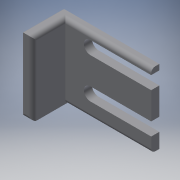
# Autodesk Inventor part: Pusher
Saved by Autodesk Inventor 2019.3 (Build 233278000, 278)
## iProperties
Created: 2020-09-18
Part Number: Pusher
Material: Generisch
Document SubType Name: Modeling
Designer: Nicolas Frick
Density: 1 g/cm^3
Appearance: Vorgabe
Author: Nicolas Frick
Autodesk Inventor part; units mm, degrees
ref_plane "YZ Plane" through (0, 0, 0) normal (1, 0, 0) x (0, 1, 0)
ref_plane "XZ Plane" through (0, 0, 0) normal (0, 1, 0) x (-1, 0, 0)
ref_plane "XY Plane" through (0, 0, 0) normal (0, 0, 1) x (1, 0, 0)
sketch "Skizze1" plane through (0, 0, 0) normal (0, 0, 1) x (1, 0, 0)
  line L0 (18, 18) -> (18, 0) construction
  line L1 (2, 18) -> (18, 18) construction
  line L2 (2, 0) -> (2, 18) construction
  line L3 (18, 0) -> (2, 0) construction
  line L4 (2, 18) -> (18, 18)
  line L5 (18, 0) -> (2, 0)
  line L6 (0.5764, 6.9713) -> (-2.7403, -18.928) construction
  circle A0 centre (14.2155, 15.0333) radius 1.2952 construction
  circle A1 centre (14.2155, 5.2246) radius 1.25 construction
  line L7 (2, 18) -> (-5.9127, 18)
  line L8 (-5.9127, 18) -> (-5.9127, 0)
  line L9 (-5.9127, 0) -> (2, 0)
  line L10 (18, 15.0333) -> (3.145, 15.0333) construction
  line L11 (18, 16.6333) -> (3.145, 16.6333)
  line L12 (3.145, 13.4333) -> (18, 13.4333)
  arc A2 (3.145, 16.6333) -> (3.145, 13.4333) centre (3.145, 15.0333) ccw
  line L13 (18, 5.2246) -> (3.145, 5.2246) construction
  line L14 (18, 6.8246) -> (3.145, 6.8246)
  line L15 (3.145, 3.6246) -> (18, 3.6246)
  arc A3 (3.145, 6.8246) -> (3.145, 3.6246) centre (3.145, 5.2246) ccw
  line L16 (-5.9127, 18) -> (18, 18)
  line L17 (18, 0) -> (-5.9127, 0)
  line L18 (-5.9127, 0) -> (-5.9127, 18)
  line L19 (18, 16.6333) -> (3.145, 16.6333)
  line L20 (18, 13.4333) -> (3.145, 13.4333)
  line L21 (18, 6.8246) -> (3.145, 6.8246)
  line L22 (18, 3.6246) -> (3.145, 3.6246)
  line L23 (18, 18) -> (18, 16.6333)
  line L24 (18, 18) -> (18, 16.6333)
  line L25 (18, 13.4333) -> (18, 6.8246)
  line L26 (18, 3.6246) -> (18, 0)
  line L27 (18, 13.4333) -> (18, 6.8246)
  line L28 (18, 3.6246) -> (18, 0)
  point P0 (0, 0)
  point P1 (10.5725, 15.0333)
  point P2 (10.5725, 5.2246)
  dimension "d0" = 2.5
  dimension "d1" = 3.2
  dimension "d2" = 3.2
  constraints: 52 end point, 11 perpendicular, 8 parallel, 4 centre point, 4 point on circle, 4 tangent, 3 collinear, 3 horizontal, 2 midpoint, 1 point on line
  measures "d0" diameter of A1
  measures "d1" diameter of A2
  measures "d2" diameter of A3
extrude "Extrusion1" add sketch "Skizze1" along normal blind 10
sketch "Skizze2" plane through (0, 0, 10) normal (0, 0, 1) x (1, 0, 0)
  line L0 (-5.9127, 0) -> (18, 0) construction
  line L1 (18, 0) -> (18, 3.6246) construction
  line L2 (18, 3.6246) -> (3.145, 3.6246) construction
  arc A0 (3.145, 6.8246) -> (3.145, 3.6246) centre (3.145, 5.2246) ccw construction
  line L3 (3.145, 6.8246) -> (18, 6.8246) construction
  line L4 (18, 6.8246) -> (18, 13.4333) construction
  line L5 (18, 13.4333) -> (3.145, 13.4333) construction
  arc A1 (3.145, 16.6333) -> (3.145, 13.4333) centre (3.145, 15.0333) ccw construction
  line L6 (3.145, 16.6333) -> (18, 16.6333) construction
  line L7 (18, 16.6333) -> (18, 18) construction
  line L8 (18, 18) -> (-5.9127, 18) construction
  line L9 (-5.9127, 18) -> (-5.9127, 0) construction
  line L10 (18, 18) -> (-5.9127, 18) projected
  line L11 (-5.9127, 0) -> (18, 0) projected
  line L12 (18, 18) -> (-3, 18)
  line L13 (-3, 18) -> (-3, 0)
  line L14 (-3, 0) -> (18, 0)
  line L15 (18, 0) -> (18, 18)
  point P0 (0, 0)
  dimension "d5" = 21
  constraints: 8 end point, 2 parallel, 1 horizontal, 1 perpendicular, 1 point on line
  measures "d5" distance of L14.end L13.end
extrude "Extrusion2" cut sketch "Skizze2" against normal blind 8
fillet "Rundung1" radius 1 7 edges at (-5.9127, 18, 5) (-3, 18, 6) (-3, 9, 10) (-5.9127, 9, 10) (-4.4563, 0, 10) (7.5, 18, 2) (7.5, 0, 2)
